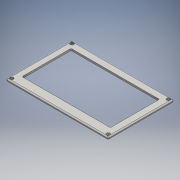
# Autodesk Inventor part: tapa
Saved by Autodesk Inventor 2016 (Build 200138000, 138)
## iProperties
Created: 2016-03-25
Part Number: tapa
Material: Generic
Document SubType Name: Modeling
Designer: Administrator
Density: 1 g/cm^3
Appearance: Default
Author: Administrator
Autodesk Inventor part; units mm, degrees
ref_plane "YZ Plane" through (0, 0, 0) normal (1, 0, 0) x (0, 1, 0)
ref_plane "XZ Plane" through (0, 0, 0) normal (0, 1, 0) x (-1, 0, 0)
ref_plane "XY Plane" through (0, 0, 0) normal (0, 0, 1) x (1, 0, 0)
sketch "Sketch1" plane through (0, 0, 0) normal (0, 0, 1) x (1, 0, 0)
  circle A0 centre (86.5, 54) radius 1.75
  circle A1 centre (-86.5, 54) radius 1.75
  circle A2 centre (86.5, -54) radius 1.75
  circle A3 centre (-86.5, -54) radius 1.75
  line L0 (91.5, 59) -> (-91.5, 59)
  line L1 (-91.5, 59) -> (-91.5, -59)
  line L2 (-91.5, -59) -> (91.5, -59)
  line L3 (91.5, -59) -> (91.5, 59)
  line L4 (78.5, -42) -> (-80, -42)
  circle A4 centre (86.5, 54) radius 1.75
  circle A5 centre (-86.5, 54) radius 1.75
  circle A6 centre (86.5, -54) radius 1.75
  circle A7 centre (-86.5, -54) radius 1.75
  line L5 (91.5, 59) -> (-91.5, 59)
  line L6 (-91.5, 59) -> (-91.5, -59)
  line L7 (-91.5, -59) -> (91.5, -59)
  line L8 (91.5, -59) -> (91.5, 59)
  line L9 (78.5, 46) -> (78.5, -42)
  line L10 (-80, -42) -> (-80, 46)
  line L11 (-128.1, 0) -> (128.1, 0) projected
  line L12 (0, -82.95) -> (0, 84.7) projected
  line L13 (-80, 46) -> (78.5, 46)
  line L14 (84.25, 60.75) -> (84.25, 59)
  line L15 (78.5, 46) -> (78.5, -42)
  line L16 (-80, -42) -> (-80, 46)
  line L17 (-84.25, 59) -> (-84.25, 60.75)
  point P0 (0, 0)
  point P1 (0, 0)
  point P2 (0, 0)
  dimension "d0" = 183
  dimension "d1" = 118
  dimension "d2" = 3.5
  dimension "d3" = 17
  dimension "d4" = 13
  dimension "d5" = 13
  dimension "d6" = 11.5
  constraints: 32 end point, 8 centre point, 2 equal radius, 2 perpendicular, 2 point on line, 2 symmetric about line
  measures "d0" distance of L0.start L0.end
  measures "d1" distance of L2.end L0.start
  measures "d2" diameter of A0
  measures "d3" distance between parallel lines of L4 L2
  measures "d4" distance between parallel lines of L13 L0
  measures "d5" distance between parallel lines of L3 L9
  measures "d6" distance between parallel lines of L1 L10
extrude "Extrusion1" add sketch "Sketch1" along normal blind 3.5 contours L3 L11 L9 L13 L12 L0 | L3 L2 L12 L4 L9 L11 | L12 L13 L10 L11 L1 L0 | L2 L1 L11 L10 L4 L12
sketch "Sketch2" plane through (0, 0, 3.5) normal (0, 0, 1) x (1, 0, 0)
  line L0 (-80, 46) -> (78.5, 46) projected
  line L1 (78.5, 46) -> (78.5, -42) projected
  line L2 (78.5, -42) -> (-80, -42) projected
  line L3 (-80, -42) -> (-80, 46) projected
  circle A0 centre (-86.5, -54) radius 1.75 projected
  circle A1 centre (86.5, -54) radius 1.75 projected
  circle A2 centre (-86.5, 54) radius 1.75 projected
  circle A3 centre (86.5, 54) radius 1.75 projected
  line L4 (91.5, 59) -> (-91.5, 59) projected
  line L5 (-91.5, 59) -> (-91.5, -59) projected
  line L6 (-91.5, -59) -> (91.5, -59) projected
  line L7 (91.5, -59) -> (91.5, 59) projected
  circle A4 centre (86.5, 54) radius 1.75
  circle A5 centre (86.5, 54) radius 1.75
  line L8 (83.5772, 55.6875) -> (86.5, 57.375)
  line L9 (86.5, 57.375) -> (89.4228, 55.6875)
  line L10 (89.4228, 55.6875) -> (89.4228, 52.3125)
  line L11 (89.4228, 52.3125) -> (86.5, 50.625)
  line L12 (86.5, 50.625) -> (83.5772, 52.3125)
  line L13 (83.5772, 52.3125) -> (83.5772, 55.6875)
  circle A6 centre (86.5, 54) radius 3.375 construction
  line L14 (-89.4228, 52.3125) -> (-89.4228, 55.6875)
  line L15 (-89.4228, 55.6875) -> (-86.5, 57.375)
  line L16 (-86.5, 57.375) -> (-83.5772, 55.6875)
  line L17 (-83.5772, 55.6875) -> (-83.5772, 52.3125)
  line L18 (-83.5772, 52.3125) -> (-86.5, 50.625)
  line L19 (-86.5, 50.625) -> (-89.4228, 52.3125)
  line L20 (-86.5, -57.375) -> (-89.4228, -55.6875)
  line L21 (-89.4228, -55.6875) -> (-89.4228, -52.3125)
  line L22 (-89.4228, -52.3125) -> (-86.5, -50.625)
  line L23 (-86.5, -50.625) -> (-83.5772, -52.3125)
  line L24 (-83.5772, -52.3125) -> (-83.5772, -55.6875)
  line L25 (-83.5772, -55.6875) -> (-86.5, -57.375)
  line L26 (83.5772, -55.6875) -> (83.5772, -52.3125)
  line L27 (83.5772, -52.3125) -> (86.5, -50.625)
  line L28 (86.5, -50.625) -> (89.4228, -52.3125)
  line L29 (89.4228, -52.3125) -> (89.4228, -55.6875)
  line L30 (89.4228, -55.6875) -> (86.5, -57.375)
  line L31 (86.5, -57.375) -> (83.5772, -55.6875)
  point P0 (0, 0)
  point P1 (89.4228, 54)
  point P2 (-83.5772, 54)
  point P3 (-83.5772, -54)
  point P4 (89.4228, -54)
  dimension "d9" = 6.75
  dimension "d12" = 173
  dimension "d19" = 108
  constraints: 48 end point, 4 coincident, 2 centre point, 1 horizontal, 1 midpoint, 1 vertical, 1 vertical alignment, 55 other
  measures "d12" distance of L13.start L14.start
  measures "d19" distance of L18.end L20.start
extrude "Extrusion3" cut sketch "Sketch2" against normal blind 2.5 contours L8 L9 L10 L11 L12 L13 | L14 L15 L16 L17 L18 L19 | L20 L21 L22 L23 L24 L25 | L26 L27 L28 L29 L30 L31
fillet "Fillet1" radius 2 12 edges at (-91.5, -59, 1.75) (91.5, -59, 1.75) (-91.5, 59, 1.75) (91.5, 59, 1.75) (91.5, 0, 3.5) (0, 59, 3.5) (-91.5, 0, 3.5) (0, -59, 3.5) (-80, 46, 1.75) (78.5, 46, 1.75) (78.5, -42, 1.75) (-80, -42, 1.75)
body "Solid1"
